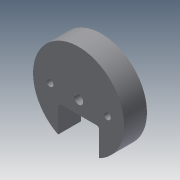
# Autodesk Inventor part: ruka_lozisko
Saved by Autodesk Inventor 2013 (Build 170138000, 138)
## iProperties
Created: 2013-05-25
Part Number: ruka_lozisko
Material: Generic
Document SubType Name: Modeling
Designer: idle-rug
Density: 1 g/cm^3
Author: idle-rug
Autodesk Inventor part; units mm, degrees
ref_plane "YZ Plane" through (0, 0, 0) normal (1, 0, 0) x (0, 1, 0)
ref_plane "XZ Plane" through (0, 0, 0) normal (0, 1, 0) x (-1, 0, 0)
ref_plane "XY Plane" through (0, 0, 0) normal (0, 0, 1) x (1, 0, 0)
sketch "Sketch1" plane through (0, 0, 0) normal (0, 1, 0) x (-1, 0, 0)
  circle A0 centre (0, 0) radius 20
  dimension "d0" = 40
  constraints: 1 centre point, 1 coincident
  measures "d0" diameter of A0
extrude "Extrusion1" add sketch "Sketch1" along normal blind 10
sketch "Sketch2" plane through (0, 10, 0) normal (0, 1, 0) x (1, 0, 0)
  circle A0 centre (0, 0) radius 20 projected
  circle A1 centre (0, 0) radius 6
  dimension "d3" = 12
  constraints: 1 centre point, 1 coincident
  measures "d3" diameter of A1
extrude "Extrusion2" cut sketch "Sketch2" against normal blind 10 contours A1
sketch "Sketch3" plane through (0, 10, 0) normal (0, 1, 0) x (1, 0, 0)
  circle A0 centre (-12.593, 0) radius 1.5
  circle A1 centre (12.593, 0) radius 1.5
  dimension "d7" = 3
  dimension "d8" = 3
  constraints: 2 centre point
  measures "d7" diameter of A0
  measures "d8" diameter of A1
extrude "Extrusion3" cut sketch "Sketch3" against normal blind 10
sketch "Sketch6" plane through (0, 10, 0) normal (0, 1, 0) x (1, 0, 0)
  circle A0 centre (0, 0) radius 6 projected
  circle A1 centre (0, 0) radius 20 projected
  circle A2 centre (0, 0) radius 5
  dimension "d11" = 10
  constraints: 1 centre point, 1 coincident
  measures "d11" diameter of A2
extrude "Extrusion4" add sketch "Sketch6" against normal blind 10 contours A0
sketch "Sketch7" plane through (0, 10, 0) normal (0, 1, 0) x (1, 0, 0)
  circle A0 centre (0, 0) radius 5 projected
  circle A1 centre (0, 0) radius 20 projected
  circle A2 centre (0, 0) radius 3
  dimension "d14" = 6
  constraints: 1 centre point, 1 coincident
  measures "d14" diameter of A2
extrude "Extrusion5" add sketch "Sketch7" against normal blind 2 contours A0
sketch "Sketch8" plane through (0, 10, 0) normal (0, 1, 0) x (1, 0, 0)
  circle A0 centre (0, 0) radius 20 projected
  line L0 (9, 17.8606) -> (9, 7.8606)
  line L1 (9, 7.8606) -> (-9, 7.8606)
  line L2 (-9, 7.8606) -> (-9, 17.8606)
  line L3 (-9, 17.8606) -> (9, 7.8606) construction
  line L4 (9, 17.8606) -> (-9, 7.8606) construction
  arc A1 (9, 17.8606) -> (-9, 17.8606) centre (0, 0) ccw
  point P0 (0, 12.8606)
  dimension "d17" = 18
  dimension "d18" = 10
  constraints: 10 end point, 4 point on circle, 2 midpoint, 1 centre point, 1 concentric, 1 parallel
  measures "d17" distance of L0.end L1.end
  measures "d18" distance of L0.start L0.end
extrude "Extrusion6" cut sketch "Sketch8" against normal blind 10 contours L0 L1 L2 A0 picked at (0, 11.9071)
sketch "Sketch9" plane through (0, 10, 0) normal (0, 1, 0) x (1, 0, 0)
  line L0 (-9, 7.8606) -> (9, 7.8606)
  line L1 (9, 7.8606) -> (9, 5.8606)
  line L2 (9, 5.8606) -> (-9, 5.8606)
  line L3 (-9, 5.8606) -> (-9, 7.8606)
  dimension "d21" = 18
  dimension "d25" = 2
  constraints: 8 end point, 2 parallel, 1 horizontal, 1 perpendicular
  measures "d21" distance of L1.end L2.end
  measures "d25" distance of L2.end L0.start
extrude "Extrusion7" cut sketch "Sketch9" against normal blind 10
sketch "Sketch10" plane through (0, 0, 0) normal (0, -1, 0) x (1, 0, 0)
  circle A0 centre (0, 0) radius 5 projected
extrude "Extrusion8" add sketch "Sketch10" against normal blind 8
sketch "Sketch11" plane through (0, 8, 0) normal (0, 1, 0) x (1, 0, 0)
  circle A0 centre (0, 0) radius 3 projected
extrude "Extrusion9" cut sketch "Sketch11" against normal blind 8
sketch "Sketch12" plane through (0, 10, 0) normal (0, 1, 0) x (1, 0, 0)
  circle A0 centre (0, 0) radius 3 projected
  arc A1 (-9, 17.8606) -> (9, 17.8606) centre (0, 0) ccw projected
  circle A2 centre (0, 0) radius 2
  dimension "d32" = 4
  constraints: 1 centre point, 1 coincident
  measures "d32" diameter of A2
extrude "Extrusion10" add sketch "Sketch12" against normal blind 10
fillet "Fillet1" radius 1 2 edges at (9, 5, -5.8606) (-9, 5, -5.8606)
body "Solid1"
